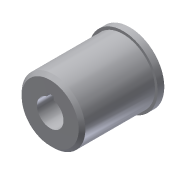
# Autodesk Inventor part: LM Colson Hub 500 key
Saved by Autodesk Inventor 2013 (Build 170138000, 138)
## iProperties
Created: 2013-07-18
Part Number: LM Colson Hub 500 key
Material: Aluminum 6061
Document SubType Name: Modeling
Designer: Nemo
Density: 1 g/cm^3
Author: Nemo
Autodesk Inventor part; units mm, degrees
ref_plane "YZ Plane" through (0, 0, 0) normal (1, 0, 0) x (0, 1, 0)
ref_plane "XZ Plane" through (0, 0, 0) normal (0, 1, 0) x (-1, 0, 0)
ref_plane "XY Plane" through (0, 0, 0) normal (0, 0, 1) x (1, 0, 0)
sketch "Sketch1" plane through (0, 0, 0) normal (0, 0, 1) x (1, 0, 0)
  circle A0 centre (0, 0) radius 15.24
  dimension "d0" = 30.48
  constraints: 1 centre point, 1 coincident
  measures "d0" diameter of A0
extrude "Extrusion1" add sketch "Sketch1" along normal mid plane 34.925
sketch "Sketch2" plane through (0, 0, -17.4625) normal (0, 0, -1) x (-1, 0, 0)
  circle A0 centre (0, 0) radius 15.24 construction
  circle A1 centre (0, 0) radius 16.51
  dimension "d5" = 33.02
  constraints: 1 centre point, 1 coincident
  measures "d5" diameter of A1
extrude "Extrusion2" add sketch "Sketch2" along normal blind 3.175
sketch "Sketch3" plane through (0, 0, 17.4625) normal (0, 0, 1) x (1, 0, 0)
  circle A0 centre (0, 0) radius 15.24 construction
  circle A1 centre (0, 0) radius 6.35
  line L0 (-1.5875, 7.7359) -> (1.5875, 7.7359)
  line L1 (1.5875, 7.7359) -> (1.5875, 4.5609)
  line L2 (1.5875, 4.5609) -> (-1.5875, 4.5609)
  line L3 (-1.5875, 4.5609) -> (-1.5875, 7.7359)
  point P0 (0, 7.7359)
  point P1 (-1.5875, 6.1484)
  dimension "d8" = 12.7
  dimension "d9" = 3.175
  dimension "d10" = 3.175
  constraints: 8 end point, 2 midpoint, 2 parallel, 1 coincident, 1 horizontal, 1 perpendicular, 1 vertical alignment, 3 other
  measures "d9" distance of L0.start L0.end
  measures "d10" distance of L2.end L0.start
extrude "Extrusion3" cut sketch "Sketch3" against normal through all
chamfer "Chamfer1" distance 1.5875 angle 45 1 edges at (-15.24, 0, 17.4625)
body "Solid1"
